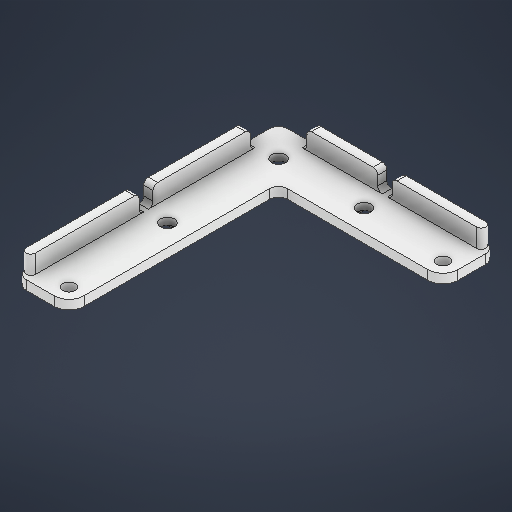
# Autodesk Inventor part: CNC-027-XAxisWireDuct
Saved by Autodesk Inventor 2026.2 (Build 302298000, 298)
## iProperties
Created: 2026-06-25
Part Number: CNC-027-XAxisWireDuct
Material: ABS Plastic
Document SubType Name: Modeling
Designer: Kenji
Density: 1.06 g/cm^3
Appearance: Smooth - White
Author: Kenji
Autodesk Inventor part; units mm, degrees
ref_plane "YZ Plane" through (0, 0, 0) normal (1, 0, 0) x (0, 1, 0)
ref_plane "XZ Plane" through (0, 0, 0) normal (0, 1, 0) x (-1, 0, 0)
ref_plane "XY Plane" through (0, 0, 0) normal (0, 0, 1) x (1, 0, 0)
sketch "Sketch1" plane through (0, 0, 0) normal (0, 1, 0) x (-1, 0, 0)
  circle A0 centre (0, 0) radius 2.1
  circle A1 centre (56.4375, 71.9375) radius 2.1
  circle A2 centre (56.4375, 71.9375) radius 5.148 construction
  circle A3 centre (0, 0) radius 5.148 construction
  line L0 (51.2895, 71.9375) -> (51.2895, 8.323)
  line L1 (48.1145, 5.148) -> (0, 5.148)
  line L2 (56.4375, 77.0855) -> (65.9625, 77.0855)
  line L3 (69.1375, 73.9105) -> (69.1375, -9.525)
  line L4 (65.9625, -12.7) -> (-1.973, -12.7)
  line L5 (-5.148, -9.525) -> (-5.148, 0)
  arc A4 (69.1375, 73.9105) -> (65.9625, 77.0855) centre (65.9625, 73.9105) ccw
  arc A5 (-5.148, -9.525) -> (-1.973, -12.7) centre (-1.973, -9.525) ccw
  arc A6 (65.9625, -12.7) -> (69.1375, -9.525) centre (65.9625, -9.525) ccw
  arc A7 (48.1145, 5.148) -> (51.2895, 8.323) centre (48.1145, 8.323) ccw
  arc A8 (56.4375, 77.0855) -> (51.2895, 71.9375) centre (56.4375, 71.9375) ccw
  arc A9 (0, 5.148) -> (-5.148, 0) centre (0, 0) ccw
  point P0 (-5.148, -12.7)
  dimension "d0" = 4.2
  dimension "d1" = 56.4375
  dimension "d2" = 71.9375
  dimension "d3" = 3.048
  dimension "d4" = 12.7
  dimension "d5" = 3.175
  dimension "d6" = 3.175
  constraints: 16 point on circle, 14 tangent, 12 end point, 10 centre point, 5 equal radius, 4 perpendicular, 2 coincident, 2 point on line, 2 vertical, 1 horizontal
  measures "d0" diameter of A0
  measures "d1" horizontal distance of point (0, 0) A1.centre
  measures "d2" vertical distance of point (0, 0) A1.centre
  measures "d3" radial gap between concentric circles of A1 A2
  measures "d4" distance of point (-5.148, -12.7) L5.end
  measures "d5" radius of A4
  measures "d6" radius of A6
extrude "Extrusion1" add sketch "Sketch1" along normal blind 3.175
sketch "Sketch2" plane through (0, 3.175, 0) normal (0, 1, 0) x (1, 0, 0)
  line L0 (-51.2895, -71.9375) -> (-51.2895, -8.323) projected
  arc A0 (-48.1145, -5.148) -> (-51.2895, -8.323) centre (-48.1145, -8.323) ccw projected
  line L1 (-48.1145, -5.148) -> (0, -5.148) projected
  arc A1 (0, -5.148) -> (5.148, 0) centre (0, 0) ccw projected
  line L2 (5.148, 0) -> (5.148, 9.525) projected
  arc A2 (5.148, 9.525) -> (1.973, 12.7) centre (1.973, 9.525) ccw projected
  line L3 (1.973, 12.7) -> (-65.9625, 12.7) projected
  arc A3 (-65.9625, 12.7) -> (-69.1375, 9.525) centre (-65.9625, 9.525) ccw projected
  line L4 (-69.1375, 9.525) -> (-69.1375, -73.9105) projected
  arc A4 (-69.1375, -73.9105) -> (-65.9625, -77.0855) centre (-65.9625, -73.9105) ccw projected
  line L5 (-65.9625, -77.0855) -> (-56.4375, -77.0855) projected
  arc A5 (-56.4375, -77.0855) -> (-51.2895, -71.9375) centre (-56.4375, -71.9375) ccw projected
  circle A6 centre (0, 0) radius 2.1 projected
  circle A7 centre (-56.4375, -71.9375) radius 2.1 projected
  line L6 (-65.9625, -73.9105) -> (-65.9625, 6.35)
  line L7 (-62.7875, 9.525) -> (1.973, 9.525)
  arc A8 (1.973, 9.525) -> (1.973, 9.525) centre (1.973, 9.525) ccw
  line L8 (1.973, 9.525) -> (1.973, 0) construction
  arc A9 (0, -1.973) -> (1.973, 0) centre (0, 0) ccw
  line L9 (0, -1.973) -> (-48.1145, -1.973) construction
  arc A10 (-48.1145, -1.973) -> (-54.4645, -8.323) centre (-48.1145, -8.323) ccw construction
  line L10 (-54.4645, -8.323) -> (-54.4645, -71.9375) construction
  arc A11 (-56.4375, -73.9105) -> (-54.4645, -71.9375) centre (-56.4375, -71.9375) ccw
  line L11 (-56.4375, -73.9105) -> (-65.9625, -73.9105) construction
  arc A12 (-62.7875, 9.525) -> (-65.9625, 6.35) centre (-62.7875, 6.35) ccw
  line L12 (-65.9625, -73.9105) -> (-65.9625, -77.0855)
  line L13 (1.973, 9.525) -> (5.148, 9.525)
  point P0 (-65.9625, 9.525)
  point P1 (1.973, 9.525)
  dimension "d9" = 3.175
  dimension "d10" = 3.175
  constraints: 16 end point, 8 point on circle, 5 centre point, 2 coincident with centre, 2 point on line, 2 tangent, 1 perpendicular, 1 vertical, 19 other
  measures "d9" distance between parallel lines of L6 L4
  measures "d10" radius of A12
sketch "Sketch2 outline for Extrusion2" plane through (0, 3.175, 0) normal (0, 1, 0) x (1, 0, 0)
  line L0 (-65.9625, -73.9105) -> (-65.9625, 6.35)
  line L1 (-65.9625, -77.0855) -> (-65.9625, -73.9105)
  arc A0 (-69.1375, -73.9105) -> (-65.9625, -77.0855) centre (-65.9625, -73.9105) ccw
  line L2 (-69.1375, 9.525) -> (-69.1375, -73.9105)
  arc A1 (-65.9625, 12.7) -> (-69.1375, 9.525) centre (-65.9625, 9.525) ccw
  line L3 (1.973, 12.7) -> (-65.9625, 12.7)
  arc A2 (5.148, 9.525) -> (1.973, 12.7) centre (1.973, 9.525) ccw
  line L4 (1.973, 9.525) -> (5.148, 9.525)
  line L5 (-62.7875, 9.525) -> (1.973, 9.525)
  arc A3 (-65.9625, 6.35) -> (-62.7875, 9.525) centre (-62.7875, 6.35) cw
extrude "Extrusion2" add sketch "Sketch2 outline for Extrusion2" along normal blind 6.35
fillet "Fillet1" radius 1.5875 2 edges at (5.148, 6.35, -9.525) (-65.9625, 6.35, 77.0855)
sketch "Sketch3" plane through (0, 3.175, 0) normal (0, 1, 0) x (1, 0, 0)
  circle A0 centre (-29.313, 2.1885) radius 2.38125
  circle A1 centre (-58.626, 2.1885) radius 2.38125
  circle A2 centre (-58.626, -35.96875) radius 2.38125
  circle A3 centre (-56.4375, -71.9375) radius 2.1
  line L0 (-65.9625, -73.9105) -> (-65.9625, 6.35)
  line L1 (-51.2895, -71.9375) -> (-51.2895, -8.323)
  line L2 (-48.1145, -5.148) -> (0, -5.148)
  point P0 (0, 0)
  dimension "d14" = 4.7625
  dimension "d15" = 71.9375
  dimension "d16" = 35.96875
  dimension "d17" = 14.673
  dimension "d18" = 7.3365
  dimension "d19" = 7.3365
  dimension "d20" = 58.626
  dimension "d21" = 29.313
  constraints: 3 centre point, 2 equal radius, 1 horizontal alignment, 1 vertical alignment
  measures "d14" diameter of A0
  measures "d15" vertical distance of point (0, 0) A3.centre
  measures "d16" vertical distance of A2.centre point (0, 0)
  measures "d17" distance between parallel lines of L0 L1
  measures "d18" distance from line of A2.centre L1
  measures "d19" distance from line of A0.centre L2
  measures "d20" horizontal distance of A2.centre point (0, 0)
  measures "d21" horizontal distance of A0.centre point (0, 0)
extrude "Extrusion3" cut sketch "Sketch3" against normal through all contours A0 | A1 | A2
sketch "Sketch4" plane through (0, 0, 0) normal (0, -1, 0) x (1, 0, 0)
  circle A0 centre (-58.626, 35.96875) radius 2.38125
  circle A1 centre (-58.626, -2.1885) radius 2.38125
  circle A2 centre (-29.313, -2.1885) radius 2.38125
  line L0 (-51.2895, 71.9375) -> (-51.2895, 8.323)
  arc A3 (-51.2895, 71.9375) -> (-56.4375, 77.0855) centre (-56.4375, 71.9375) ccw
  line L1 (-65.9625, 77.0855) -> (-56.4375, 77.0855)
  arc A4 (-65.9625, 77.0855) -> (-69.1375, 73.9105) centre (-65.9625, 73.9105) ccw
  line L2 (-69.1375, -9.525) -> (-69.1375, 73.9105)
  arc A5 (-69.1375, -9.525) -> (-65.9625, -12.7) centre (-65.9625, -9.525) ccw
  line L3 (1.973, -12.7) -> (-65.9625, -12.7)
  arc A6 (1.973, -12.7) -> (5.148, -9.525) centre (1.973, -9.525) ccw
  line L4 (5.148, 0) -> (5.148, -9.525)
  arc A7 (5.148, 0) -> (0, 5.148) centre (0, 0) ccw
  line L5 (-48.1145, 5.148) -> (0, 5.148)
  arc A8 (-51.2895, 8.323) -> (-48.1145, 5.148) centre (-48.1145, 8.323) ccw
  circle A9 centre (0, 0) radius 2.1
  circle A10 centre (-56.4375, 71.9375) radius 2.1
  line L6 (-58.626, 33.5875) -> (-69.1375, 33.5875)
  line L7 (-58.626, 38.35) -> (-69.1375, 38.35)
  line L8 (-58.626, 0.19275) -> (-69.1375, 0.19275)
  line L9 (-56.24475, -2.1885) -> (-56.24475, -12.7)
  circle A11 centre (-58.626, 35.96875) radius 2.38125
  line L10 (-26.93175, -2.1885) -> (-26.93175, -12.7)
  line L11 (-31.69425, -2.1885) -> (-31.69425, -12.7)
  constraints: 12 end point, 6 perpendicular, 6 point on circle, 6 point on line, 6 tangent
extrude "Extrusion4" cut sketch "Sketch4" against normal blind 0.79375 contours A0 L6 L2 L7 | L8 A1 L9 L3 A5 L2 | L11 A2 L10 L3
sketch "Sketch5" plane through (0, 9.525, 0) normal (0, 1, 0) x (1, 0, 0)
  arc A0 (-69.1375, -73.9105) -> (-65.9625, -73.9105) centre (-67.55, -73.9105) ccw
  line L0 (-65.9625, -73.9105) -> (-65.9625, 6.35)
  arc A1 (-62.7875, 9.525) -> (-65.9625, 6.35) centre (-62.7875, 6.35) ccw
  line L1 (-62.7875, 9.525) -> (1.973, 9.525)
  arc A2 (1.973, 9.525) -> (1.973, 12.7) centre (1.973, 11.1125) ccw
  line L2 (1.973, 12.7) -> (-65.9625, 12.7)
  arc A3 (-65.9625, 12.7) -> (-69.1375, 9.525) centre (-65.9625, 9.525) ccw
  line L3 (-69.1375, 9.525) -> (-69.1375, -73.9105)
  line L4 (-56.24475, 1.903056) -> (-56.24475, 12.7)
  circle A4 centre (-58.626, 2.1885) radius 2.38125
  line L5 (-58.626, -0.19275) -> (-69.1375, -0.19275)
  circle A5 centre (-58.626, -35.96875) radius 2.38125
  circle A6 centre (-58.626, 2.1885) radius 2.38125
  circle A7 centre (-29.313, 2.1885) radius 2.38125
  circle A8 centre (-56.4375, -71.9375) radius 2.1
  circle A9 centre (0, 0) radius 2.1
  line L6 (1.973, 9.525) -> (-62.7875, 9.525)
  arc A10 (-62.7875, 9.525) -> (-65.9625, 6.35) centre (-62.7875, 6.35) ccw
  line L7 (-65.9625, 6.35) -> (-65.9625, -73.9105)
  arc A11 (-69.1375, -73.9105) -> (-65.9625, -73.9105) centre (-67.55, -73.9105) ccw
  arc A12 (-69.1375, -73.9105) -> (-65.9625, -77.0855) centre (-65.9625, -73.9105) ccw
  line L8 (-65.9625, -77.0855) -> (-56.4375, -77.0855)
  arc A13 (-56.4375, -77.0855) -> (-51.2895, -71.9375) centre (-56.4375, -71.9375) ccw
  line L9 (-51.2895, -71.9375) -> (-51.2895, -8.323)
  arc A14 (-48.1145, -5.148) -> (-51.2895, -8.323) centre (-48.1145, -8.323) ccw
  line L10 (-48.1145, -5.148) -> (0, -5.148)
  arc A15 (0, -5.148) -> (5.148, 0) centre (0, 0) ccw
  line L11 (5.148, 0) -> (5.148, 9.525)
  arc A16 (5.148, 9.525) -> (1.973, 12.7) centre (1.973, 9.525) ccw
  arc A17 (1.973, 9.525) -> (1.973, 12.7) centre (1.973, 11.1125) ccw
  line L12 (-31.693284, 2.120672) -> (-31.99475, 12.7)
  line L13 (-26.93175, 2.1885) -> (-26.93175, 12.7)
  line L14 (-58.626, -33.5875) -> (-69.1375, -33.5875)
  line L15 (-58.626, -38.35) -> (-69.1375, -38.35)
  point P0 (-56.24475, 2.1885)
  constraints: 12 end point, 5 perpendicular, 5 point on line, 4 point on circle, 4 tangent, 1 horizontal, 1 midpoint, 1 vertical, 2 other
extrude "Extrusion5" cut sketch "Sketch5" against normal up to surface (6.35 mm away) contours L3 L14 L0 L15 | L0 L14 A5 L15 | L3 A3 L2 L4 L1 A1 L0 L5 | L0 A1 L1 L4 A4 L5 | L2 L13 L1 L12 | L1 L13 A7 L12
fillet "Fillet2" radius 1.5875 12 edges at (-67.55, 9.525, 33.5875) (-67.55, 3.175, 33.5875) (-67.55, 9.525, 38.35) (-67.55, 3.175, 38.35) (-56.2448, 3.175, -11.1125) (-56.2448, 9.525, -11.1125) (-67.55, 3.175, 0.1928) (-67.55, 9.525, 0.1928) (-26.9318, 9.525, -11.1125) (-26.9318, 3.175, -11.1125) (-31.9495, 9.525, -11.1125) (-31.9495, 3.175, -11.1125)
equation "\"d16\" = 0.5 * d15"
equation "\"d18\" = 0.5 * d17"
equation "\"d19\" = d18"
equation "\"d21\" = 0.5 * d20"
body "Solid1"
